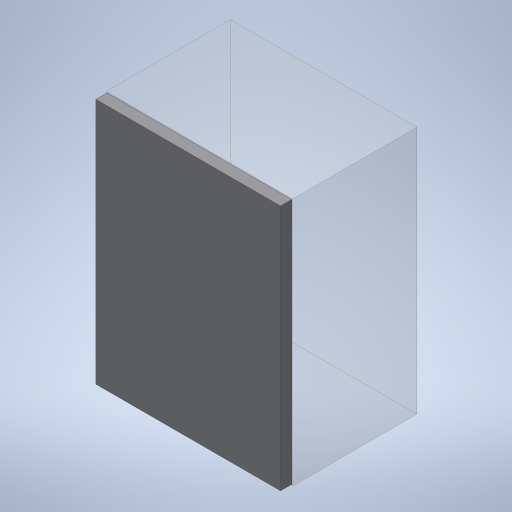
# Autodesk Inventor part: Laminated Board Skeleton
Saved by Autodesk Inventor 2024 (Build 280153000, 153)
## iProperties
RuleStatus: InUse
Created: 2014-05-07
Part Number: Laminated Board Skeleton
Material: Generic
Document SubType Name: Modeling
Designer: SauliusD
Density: 1 g/cm^3
Appearance: Default
Description: Laminated Board Facade Skeleton
Author: SauliusD
Autodesk Inventor part; units mm, degrees
ref_plane "YZ Plane" through (0, 0, 0) normal (1, 0, 0) x (0, 1, 0)
ref_plane "XZ Plane" through (0, 0, 0) normal (0, 1, 0) x (-1, 0, 0)
ref_plane "XY Plane" through (0, 0, 0) normal (0, 0, 1) x (1, 0, 0)
sketch "Sketch2" plane through (0, 0, 0) normal (0, 1, 0) x (-1, 0, 0)
  line L0 (150, -200) -> (-150, -200)
  line L1 (-150, -200) -> (-150, 200)
  line L2 (-150, 200) -> (150, 200)
  line L3 (150, 200) -> (150, -200)
  line L4 (150, -200) -> (-150, 200) construction
  line L5 (-150, -200) -> (150, 200) construction
  point P0 (0, 0)
  dimension "Width" = 300
  dimension "Height" = 400
  constraints: 12 end point, 2 midpoint, 2 parallel, 1 horizontal, 1 perpendicular
  measures "Width" distance of L1.end L2.end
  measures "Height" distance of L0.end L1.end
sketch "Sketch1" plane through (0, 0, 0) normal (0, 1, 0) x (-1, 0, 0)
  line L0 (148.5, -198.5) -> (-148.5, -198.5)
  line L1 (-148.5, -198.5) -> (-148.5, 198.5)
  line L2 (-148.5, 198.5) -> (148.5, 198.5)
  line L3 (148.5, 198.5) -> (148.5, -198.5)
  line L4 (-150, 200) -> (150, 200) construction
  line L5 (150, 200) -> (150, -200) construction
  line L6 (150, -200) -> (-150, -200) construction
  line L7 (-150, -200) -> (-150, 200) construction
  point P0 (0, 0)
  dimension "Off_From_Top" = 1.5
  dimension "Off_From_Left" = 1.5
  dimension "Off_From_Bottom" = 1.5
  dimension "Off_From_Right" = 1.5
  constraints: 8 end point, 2 parallel, 1 horizontal, 1 perpendicular
  measures "Off_From_Top" distance between parallel lines of L4 L2
  measures "Off_From_Left" distance between parallel lines of L5 L3
  measures "Off_From_Bottom" distance between parallel lines of L6 L0
  measures "Off_From_Right" distance between parallel lines of L7 L1
extrude "Extrusion1" add sketch "Sketch1" against normal blind 18
extrude "Extrusion2" add sketch "Sketch2" along normal blind 200 separate body
equation "\"Total_Offset\" = 0.001"
equation "\"Hinge_Gap\" = 0"
equation "\"Inset_Dist\" = 0"
body "Solid1"
body "Solid2"
